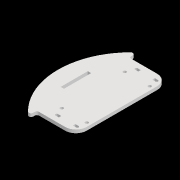
# Autodesk Inventor part: Parte inferior 2
Saved by Autodesk Inventor 2022 (Build 260153000, 153)
## iProperties
Created: 2021-09-27
Part Number: Parte inferior 2
Material: Genérico
Document SubType Name: Modeling
Designer: Julio R
Density: 1 g/cm^3
Appearance: Valor por defecto
Author: Julio R
Autodesk Inventor part; units mm, degrees
ref_plane "YZ Plane" through (0, 0, 0) normal (1, 0, 0) x (0, 1, 0)
ref_plane "XZ Plane" through (0, 0, 0) normal (0, 1, 0) x (-1, 0, 0)
ref_plane "XY Plane" through (0, 0, 0) normal (0, 0, 1) x (1, 0, 0)
sketch "Boceto1" plane through (0, 0, 0) normal (0, 1, 0) x (-1, 0, 0)
  line L0 (3, 0) -> (33, 0)
  line L1 (36, -3) -> (36, -62)
  line L2 (33, -65) -> (3, -65)
  line L3 (0, -62) -> (0, -3)
  circle A0 centre (3.5, -61.5) radius 1.375
  arc A1 (36, -3) -> (33, 0) centre (33, -3) ccw
  arc A2 (3, 0) -> (0, -3) centre (3, -3) ccw
  arc A3 (0, -62) -> (3, -65) centre (3, -62) ccw
  arc A4 (33, -65) -> (36, -62) centre (33, -62) ccw
  circle A5 centre (26.5, -61.5) radius 1.375
  circle A6 centre (3.5, -3.5) radius 1.375
  circle A7 centre (26.5, -3.5) radius 1.375
  line L4 (36, 0) -> (0, 0)
  line L5 (0, 0) -> (0, 10)
  line L6 (0, 10) -> (36, 10)
  line L7 (36, 10) -> (36, 0)
  line L8 (36, -65) -> (0, -65)
  line L9 (0, -65) -> (0, -75)
  line L10 (0, -75) -> (36, -75)
  line L11 (36, -75) -> (36, -65)
  line L12 (7.5, 0) -> (20.5, 0)
  line L13 (20.5, 0) -> (20.5, 10)
  line L14 (20.5, 10) -> (7.5, 10)
  line L15 (7.5, 10) -> (7.5, 0)
  line L16 (7.5, 0) -> (20.5, 10) construction
  line L17 (20.5, 0) -> (7.5, 10) construction
  line L18 (7.5, -75) -> (20.5, -75)
  line L19 (20.5, -75) -> (20.5, -65)
  line L20 (20.5, -65) -> (7.5, -65)
  line L21 (7.5, -65) -> (7.5, -75)
  line L22 (7.5, -75) -> (20.5, -65) construction
  line L23 (20.5, -75) -> (7.5, -65) construction
  line L24 (36, -32.5) -> (0, -32.5)
  line L25 (36, 0) -> (36, -3)
  line L26 (0, 0) -> (0, -3)
  line L27 (0, -62) -> (0, -65)
  line L28 (36, -62) -> (36, -65)
  line L29 (36, -22.5) -> (49, -22.5)
  line L30 (49, -22.5) -> (49, -42.5)
  line L31 (49, -42.5) -> (36, -42.5)
  line L32 (36, -42.5) -> (36, -22.5)
  arc A8 (49, -42.5) -> (49, -22.5) centre (49, -32.5) ccw
  line L33 (20.5, 5.3) -> (23.5, 5.3)
  line L34 (23.5, 5.3) -> (23.5, 3)
  line L35 (23.5, 3) -> (20.5, 3)
  line L36 (20.5, 3) -> (20.5, 5.3)
  arc A9 (23.5, 3) -> (23.5, 5.3) centre (23.5, 4.15) ccw
  line L37 (14, 0) -> (14, -65)
  line L38 (7.5, 5.3) -> (4.5, 5.3)
  line L39 (4.5, 5.3) -> (4.5, 3)
  line L40 (4.5, 3) -> (7.5, 3)
  line L41 (7.5, 3) -> (7.5, 5.3)
  arc A10 (4.5, 5.3) -> (4.5, 3) centre (4.5, 4.15) ccw
  line L42 (20.5, -70.3) -> (23.5, -70.3)
  line L43 (23.5, -70.3) -> (23.5, -68)
  line L44 (23.5, -68) -> (20.5, -68)
  line L45 (20.5, -68) -> (20.5, -70.3)
  arc A11 (23.5, -70.3) -> (23.5, -68) centre (23.5, -69.15) ccw
  line L46 (4.5, -68) -> (7.5, -68)
  arc A12 (4.5, -68) -> (4.5, -70.3) centre (4.5, -69.15) ccw
  line L47 (7.5, -70.3) -> (4.5, -70.3)
  line L48 (4.5, -70.3) -> (4.5, -68)
  line L49 (7.5, -68) -> (7.5, -70.3)
  line L50 (36, 0) -> (49, 0)
  line L51 (49, 0) -> (49, -65)
  line L52 (49, -65) -> (36, -65)
  line L53 (36, -65) -> (36, 0)
  line L54 (44, -20) -> (41, -20)
  line L55 (41, -20) -> (41, -45)
  line L56 (41, -45) -> (44, -45)
  line L57 (44, -45) -> (44, -20)
  line L58 (36, 10) -> (36, 18)
  line L59 (36, -75) -> (36, -83)
  arc A13 (36, -83) -> (36, 18) centre (-7.9402, -32.5) ccw
  line L60 (0, -75) -> (-8, -75)
  line L61 (-8, -75) -> (-8, 10)
  line L62 (-8, 10) -> (0, 10)
  line L63 (0, 10) -> (0, -75)
  line L64 (-8, 10) -> (-8, 17.5724)
  line L65 (-8, -75) -> (-8, -82.5724)
  arc A14 (-8, 17.5724) -> (-8, -82.5724) centre (14, -32.5) ccw
  point P0 (14, 5)
  point P1 (14, -70)
  point P2 (36, -42.5)
  point P3 (7.5, -70.3)
  point P4 (20.5, -70.3)
  point P5 (7.5, 5.3)
  point P6 (20.5, 3)
  point P7 (44, -32.5)
  point P8 (36, -65)
  point P9 (44, -42.5)
  point P10 (41, -42.5)
  point P11 (41, -22.5)
  point P12 (44, -22.5)
  point P13 (49, -22.5)
  point P14 (59, -32.5)
  dimension "d0" = 36
  dimension "d1" = 65
  dimension "d2" = 2.75
  dimension "d3" = 3
  dimension "d4" = 3
  dimension "d5" = 3
  dimension "d6" = 3
  dimension "d7" = 3.5
  dimension "d8" = 3.5
  dimension "d11" = 23
  dimension "d14" = 58
  dimension "d17" = 10
  dimension "d18" = 10
  dimension "d19" = 13
  dimension "d20" = 10
  dimension "d21" = 13
  dimension "d22" = 10
  dimension "d26" = 7.5
  dimension "d30" = 20
  dimension "d31" = 13
  dimension "d32" = 3
  dimension "d33" = 2.3
  dimension "d34" = 3
  dimension "d35" = 1.15
  dimension "d36" = 13
  dimension "d37" = 3
  dimension "d38" = 25
  dimension "d39" = 5
  dimension "d42" = 8
  dimension "d43" = 8
  dimension "d46" = 8
  dimension "d47" = 54.6923
  constraints: 132 end point, 23 parallel, 23 point on circle, 15 centre point, 15 symmetric about line, 15 tangent, 12 midpoint, 11 horizontal, 11 point on line, 10 perpendicular, 6 vertical, 3 collinear, 2 horizontal alignment, 9 other
  measures "d0" distance of L8.start point (0, -65)
  measures "d1" distance of L4.start L8.start
  measures "d2" diameter of A0
  measures "d3" radius of A1
  measures "d4" radius of A2
  measures "d5" radius of A3
  measures "d6" radius of A4
  measures "d7" distance from line of L3 A0.centre
  measures "d8" distance from line of L2 A0.centre
  measures "d11" distance of A0.centre A5.centre
  measures "d14" distance of A0.centre A6.centre
  measures "d17" distance of L4.end L5.end
  measures "d18" distance of L9.end L8.end
  measures "d19" distance of L14.end L13.end
  measures "d20" distance of L13.end L12.end
  measures "d21" distance of L19.end L20.end
  measures "d22" distance of L18.end L19.end
  measures "d26" distance of point (0, 0) L12.start
  measures "d30" distance between parallel lines of L31 L29
  measures "d31" distance of L29.start L29.end
  measures "d32" distance of L34.end L35.end
  measures "d33" distance of L33.end L34.end
  measures "d34" distance between parallel lines of L0 L35
  measures "d35" radius of A9
  measures "d36" distance from line of L4.start L51
  measures "d37" distance of L56.end L55.end
  measures "d38" distance of L55.end L54.end
  measures "d39" distance between parallel lines of L1 L55
  measures "d42" distance of L6.end L58.end
  measures "d43" distance of L10.end L59.end
  measures "d46" distance of L61.end L62.end
  measures "d47" radius of A14
extrude "Extrusión1" add sketch "Boceto1" along normal blind 3 contours L4 L5 L6 L15 L38 A10 L40 L0 | L0 L37 L24 L3 A2 | A2 L26 L4 | L15 L6 L13 L0 | L0 A1 L1 L24 L37 | L24 L37 L2 A3 L3 | L13 L35 A9 L33 L6 L7 L4 L0 | L24 L1 A4 L2 L37 | A3 L8 L27 | L4 L25 A1 | L1 L29 L55 L31 | L2 L19 L10 L21 | L2 L21 L46 A12 L47 L10 L9 L8 | L25 L50 L51 L29 L57 L54 L55 L1 | L7 L58 A13 A8 L51 L50 | L31 L55 L56 L57 L51 L52 L28 L1 | L2 L8 L11 L10 L19 L42 A11 L44 | L29 L57 L31 L55 | L28 L8 A4 | L30 L31 L57 L29 | A8 L30 | L52 L51 A8 A13 L59 L11
fillet "Empalme1" radius 10 2 edges at (0, 1.5, -75) (0, 1.5, 10)
extrude "Extrusión2" cut sketch "Boceto1" along normal blind 3 contours L29 L57 L31 L55
fillet "Empalme2" radius 2 4 edges at (-36, 1.5, -83) (-36, 1.5, 18) (-36, 1.5, 10) (-36, 1.5, -75)
extrude "Extrusión3" add sketch "Boceto1" along normal blind 3 contours L4 L5 L6 L15 L38 A10 L40 L0 | L3 L27 L9 L60 L61 L62 L5 L26 | L61 L65 A14 L64 | L2 L21 L46 A12 L47 L10 L9 L8
equation "\"d18\" = d17"
equation "\"d21\" = d19"
equation "\"d22\" = d20"
equation "\"d36\" = d31"
